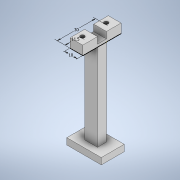
# Autodesk Inventor part: sucrose training holder
Saved by Autodesk Inventor 2020.1 (Build 241239000, 239)
## iProperties
Created: 2019-07-30
Part Number: sucrose training holder
Material: 일반
Document SubType Name: Modeling
Designer: Chang Ko
Mass: 7.19 g
Surface Area: 37.34 cm^2
Volume: 7.19 cm^3
Density: 1 g/cm^3
Appearance: 기본값
Author: Chang Ko
Autodesk Inventor part; units mm, degrees
ref_plane "YZ Plane" through (0, 0, 0) normal (1, 0, 0) x (0, 1, 0)
ref_plane "XZ Plane" through (0, 0, 0) normal (0, 1, 0) x (-1, 0, 0)
ref_plane "XY Plane" through (0, 0, 0) normal (0, 0, 1) x (1, 0, 0)
sketch "스케치1" plane through (0, 0, 0) normal (0, 1, 0) x (-1, 0, 0)
  line L0 (13.5, 9) -> (-13.5, 9)
  line L1 (-13.5, 9) -> (-13.5, -9)
  line L2 (-13.5, -9) -> (13.5, -9)
  line L3 (13.5, -9) -> (13.5, 9)
  point P0 (0, 0)
  dimension "d0" = 27
  dimension "d1" = 18
  dimension "d2" = 9
  dimension "d3" = 13.5
  constraints: 8 end point, 2 parallel, 1 horizontal, 1 perpendicular
  measures "d0" distance of L2.end L1.end
  measures "d1" distance of L1.end L0.end
  measures "d2" distance from line of point (0, 0) L0
  measures "d3" distance from line of L3 point (0, 0)
extrude "돌출1" add sketch "스케치1" along normal blind 5
sketch "스케치2" plane through (0, 5, 0) normal (0, 1, 0) x (1, 0, 0)
  line L0 (-5, -3.5) -> (5, -3.5)
  line L1 (5, -3.5) -> (5, 3.5)
  line L2 (5, 3.5) -> (-5, 3.5)
  line L3 (-5, 3.5) -> (-5, -3.5)
  line L4 (-13.5, -9) -> (13.5, -9) projected
  line L5 (-13.5, 9) -> (-13.5, -9) projected
  point P0 (0, 0)
  dimension "d6" = 10
  dimension "d7" = 7
  dimension "d8" = 5.5
  dimension "d9" = 8.5
  constraints: 8 end point, 1 horizontal, 1 parallel, 1 perpendicular, 1 vertical
  measures "d6" distance of L2.end L1.end
  measures "d7" distance of L1.end L0.end
  measures "d8" distance between parallel lines of L0 L4
  measures "d9" distance between parallel lines of L3 L5
extrude "돌출2" add sketch "스케치2" along normal blind 68
sketch "스케치3" plane through (0, 73, 0) normal (0, 1, 0) x (1, 0, 0)
  line L0 (5, 15) -> (-5, 15)
  line L1 (-5, 15) -> (-5, -15)
  line L2 (-5, -15) -> (5, -15)
  line L3 (5, -15) -> (5, 15)
  line L4 (5, 3.5) -> (-5, 3.5) projected
  line L5 (-5, 3.5) -> (-5, -3.5) projected
  line L6 (-5, -3.5) -> (5, -3.5) projected
  line L7 (5, -3.5) -> (5, 3.5) projected
  line L8 (5, 3.5) -> (-5, 3.5) projected
  line L9 (-5, 3.5) -> (-5, -3.5) projected
  point P0 (0, 0)
  dimension "d12" = 10
  dimension "d13" = 30
  dimension "d14" = 11.5
  constraints: 8 end point, 3 parallel, 1 collinear, 1 horizontal, 1 perpendicular
  measures "d12" distance of L2.end L1.end
  measures "d13" distance of L1.end L0.end
  measures "d14" distance between parallel lines of L6 L2
extrude "돌출3" add sketch "스케치3" along normal blind 2
sketch "스케치4" plane through (0, 75, 0) normal (0, 1, 0) x (1, 0, 0)
  point P0 (0, 0)
sketch "스케치5" plane through (0, 73, 0) normal (0, -1, 0) x (1, 0, 0)
  line L0 (-5, 3.5) -> (5, 3.5) projected
  line L1 (5, 15) -> (5, 3.5) projected
  line L2 (-5, 15) -> (5, 15) projected
  line L3 (-5, 3.5) -> (-5, 15) projected
  line L4 (5, -3.5) -> (-5, -3.5) projected
  line L5 (-5, -15) -> (-5, -3.5) projected
  line L6 (5, -15) -> (-5, -15) projected
  line L7 (5, -3.5) -> (5, -15) projected
  point P0 (0, 0)
sketch "스케치6" plane through (0, 75, 0) normal (0, 1, 0) x (1, 0, 0)
  line L0 (-5, 15) -> (-5, 3.5) projected
  point P0 (0, 0)
sketch "스케치7" plane through (0, 75, 0) normal (0, 1, 0) x (1, 0, 0)
  line L0 (5, 3.5) -> (5, 15) projected
  line L1 (-5, 3.5) -> (5, 3.5) projected
  line L2 (5, 15) -> (-5, 15)
  line L3 (-5, 15) -> (-5, 3.5)
  line L4 (-5, 3.5) -> (5, 3.5)
  line L5 (5, 3.5) -> (5, 15)
  line L6 (-5, -3.5) -> (-5, -15) projected
  line L7 (-5, -15) -> (5, -15) projected
  line L8 (-5, -3.5) -> (5, -3.5)
  line L9 (5, -3.5) -> (5, -15)
  line L10 (5, -15) -> (-5, -15)
  line L11 (-5, -15) -> (-5, -3.5)
  point P0 (0, 0)
  constraints: 16 end point, 4 parallel, 2 horizontal, 2 perpendicular
extrude "돌출4" add sketch "스케치7" along normal blind 5
sketch "스케치11" plane through (0, 80, 0) normal (0, 1, 0) x (1, 0, 0)
  line L0 (-5, -3.5) -> (-5, -15) projected
  line L1 (-5, -15) -> (5, -15) projected
  line L2 (5, 15) -> (-5, 15) projected
  line L3 (-5, 15) -> (-5, 3.5) projected
  point P0 (0, 0)
  point P1 (-1, -9.3)
  point P2 (-1, 9.3)
  dimension "d37" = 4
  dimension "d38" = 5.7
  dimension "d39" = 5.7
  dimension "d40" = 4
  measures "d37" distance from line of L0 point (-1, -9.3)
  measures "d38" distance from line of L1 point (-1, -9.3)
  measures "d39" distance from line of L2 point (-1, 9.3)
  measures "d40" distance from line of L3 point (-1, 9.3)
hole "구멍1" at (-1, 80, 9.3) at (-1, 80, -9.3) direction (0, -1, 0) diameter 3.242 depth 11.8 tip angle 118 thread size "M4x0.7" class "6H" standard "ANSI Metric M Profile"
